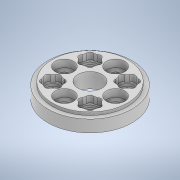
# Autodesk Inventor part: Inner_support_stand
Saved by Autodesk Inventor 2020 (Build 240168000, 168)
## iProperties
Created: 2021-09-25
Part Number: Inner_support_stand
Material: アルミニウム 2014-T4
Document SubType Name: Modeling
Designer: Masato Kubotera
Density: 2.8 g/cm^3
Appearance: 滑らか - 淡い灰色
Mass: 5.51581 g
Surface Area: 21.3058 cm^2
Volume: 1.96993 cm^3
Description: A2017 T5
Author: Masato Kubotera
Autodesk Inventor part; units mm, degrees
ref_plane "YZ Plane" through (0, 0, 0) normal (1, 0, 0) x (0, 1, 0)
ref_plane "XZ Plane" through (0, 0, 0) normal (0, 1, 0) x (-1, 0, 0)
ref_plane "XY Plane" through (0, 0, 0) normal (0, 0, 1) x (1, 0, 0)
derived "Inner_flange.ipt"
sketch "スケッチ1" plane through (0, 0, 0) normal (0, 0, 1) x (1, 0, 0)
  circle A0 centre (0, 0) radius 13.95
  line L0 (0, 13.95) -> (0, -13.95) construction
  circle A1 centre (0, 8.5) radius 1.35
  circle A2 centre (-8.5, 0) radius 1.35
  circle A3 centre (0, -8.5) radius 1.35
  circle A4 centre (8.5, 0) radius 1.35
  circle A5 centre (0, 0) radius 5 construction
  circle A6 centre (0, 0) radius 5.01
  circle A7 centre (-6.1872, 6.1872) radius 2.25
  line L1 (-9.8641, 9.8641) -> (9.8641, -9.8641) construction
  circle A8 centre (-6.1872, 6.1872) radius 1.55
  line L2 (-9.2656, 5.3623) -> (-8.9938, 6.3766) construction
  line L3 (-8.4407, 8.4407) -> (-7.4265, 8.7125) construction
  line L4 (-5.3623, 9.2656) -> (-4.6199, 8.5231) construction
  line L5 (-3.1088, 7.012) -> (-3.3806, 5.9978) construction
  line L6 (-3.9337, 3.9337) -> (-4.9479, 3.6619) construction
  line L7 (-7.012, 3.1088) -> (-7.7545, 3.8513) construction
  circle A9 centre (0, 0) radius 12.49
  arc A10 (-7.4265, 8.7125) -> (-8.7125, 7.4265) centre (-7.6983, 7.6983) ccw
  arc A11 (-8.9938, 6.3766) -> (-8.5231, 4.6199) centre (-8.2513, 5.6341) ccw
  arc A12 (-7.7545, 3.8513) -> (-5.9978, 3.3806) centre (-6.7403, 4.123) ccw
  arc A13 (-4.9479, 3.6619) -> (-3.6619, 4.9479) centre (-4.6761, 4.6761) ccw
  arc A14 (-3.3806, 5.9978) -> (-3.8513, 7.7545) centre (-4.123, 6.7403) ccw
  arc A15 (-4.6199, 8.5231) -> (-6.3766, 8.9938) centre (-5.6341, 8.2513) ccw
  line L8 (-6.3766, 8.9938) -> (-5.3623, 9.2656) construction
  line L9 (-7.4265, 8.7125) -> (-6.3766, 8.9938)
  line L10 (-4.6199, 8.5231) -> (-3.8513, 7.7545)
  line L11 (-3.8513, 7.7545) -> (-3.1088, 7.012) construction
  line L12 (-3.3806, 5.9978) -> (-3.6619, 4.9479)
  line L13 (-3.6619, 4.9479) -> (-3.9337, 3.9337) construction
  line L14 (-4.9479, 3.6619) -> (-5.9978, 3.3806)
  line L15 (-5.9978, 3.3806) -> (-7.012, 3.1088) construction
  line L16 (-7.7545, 3.8513) -> (-8.5231, 4.6199)
  line L17 (-8.5231, 4.6199) -> (-9.2656, 5.3623) construction
  line L18 (-8.9938, 6.3766) -> (-8.7125, 7.4265)
  line L19 (-8.7125, 7.4265) -> (-8.4407, 8.4407) construction
  circle A16 centre (-8.5, 0) radius 3.05
  line L20 (-8.7125, -7.4265) -> (-8.9938, -6.3766)
  circle A17 centre (-6.1872, -6.1872) radius 2.25
  circle A18 centre (-6.1872, -6.1872) radius 1.55
  circle A19 centre (0, -8.5) radius 3.05
  arc A20 (-3.8513, -7.7545) -> (-3.3806, -5.9978) centre (-4.123, -6.7403) ccw
  line L21 (-3.6619, -4.9479) -> (-3.3806, -5.9978)
  arc A21 (-3.6619, -4.9479) -> (-4.9479, -3.6619) centre (-4.6761, -4.6761) ccw
  line L22 (-5.9978, -3.3806) -> (-4.9479, -3.6619)
  arc A22 (-5.9978, -3.3806) -> (-7.7545, -3.8513) centre (-6.7403, -4.123) ccw
  line L23 (-8.5231, -4.6199) -> (-7.7545, -3.8513)
  arc A23 (-8.5231, -4.6199) -> (-8.9938, -6.3766) centre (-8.2513, -5.6341) ccw
  arc A24 (-8.7125, -7.4265) -> (-7.4265, -8.7125) centre (-7.6983, -7.6983) ccw
  line L24 (-6.3766, -8.9938) -> (-7.4265, -8.7125)
  arc A25 (-6.3766, -8.9938) -> (-4.6199, -8.5231) centre (-5.6341, -8.2513) ccw
  line L25 (-3.8513, -7.7545) -> (-4.6199, -8.5231)
  line L26 (7.4265, -8.7125) -> (6.3766, -8.9938)
  circle A26 centre (6.1872, -6.1872) radius 2.25
  circle A27 centre (6.1872, -6.1872) radius 1.55
  circle A28 centre (8.5, 0) radius 3.05
  arc A29 (7.7545, -3.8513) -> (5.9978, -3.3806) centre (6.7403, -4.123) ccw
  line L27 (4.9479, -3.6619) -> (5.9978, -3.3806)
  arc A30 (4.9479, -3.6619) -> (3.6619, -4.9479) centre (4.6761, -4.6761) ccw
  line L28 (3.3806, -5.9978) -> (3.6619, -4.9479)
  arc A31 (3.3806, -5.9978) -> (3.8513, -7.7545) centre (4.123, -6.7403) ccw
  line L29 (4.6199, -8.5231) -> (3.8513, -7.7545)
  arc A32 (4.6199, -8.5231) -> (6.3766, -8.9938) centre (5.6341, -8.2513) ccw
  arc A33 (7.4265, -8.7125) -> (8.7125, -7.4265) centre (7.6983, -7.6983) ccw
  line L30 (8.9938, -6.3766) -> (8.7125, -7.4265)
  arc A34 (8.9938, -6.3766) -> (8.5231, -4.6199) centre (8.2513, -5.6341) ccw
  line L31 (7.7545, -3.8513) -> (8.5231, -4.6199)
  line L32 (8.7125, 7.4265) -> (8.9938, 6.3766)
  circle A35 centre (6.1872, 6.1872) radius 2.25
  circle A36 centre (6.1872, 6.1872) radius 1.55
  circle A37 centre (0, 8.5) radius 3.05
  arc A38 (3.8513, 7.7545) -> (3.3806, 5.9978) centre (4.123, 6.7403) ccw
  line L33 (3.6619, 4.9479) -> (3.3806, 5.9978)
  arc A39 (3.6619, 4.9479) -> (4.9479, 3.6619) centre (4.6761, 4.6761) ccw
  line L34 (5.9978, 3.3806) -> (4.9479, 3.6619)
  arc A40 (5.9978, 3.3806) -> (7.7545, 3.8513) centre (6.7403, 4.123) ccw
  line L35 (8.5231, 4.6199) -> (7.7545, 3.8513)
  arc A41 (8.5231, 4.6199) -> (8.9938, 6.3766) centre (8.2513, 5.6341) ccw
  arc A42 (8.7125, 7.4265) -> (7.4265, 8.7125) centre (7.6983, 7.6983) ccw
  line L36 (6.3766, 8.9938) -> (7.4265, 8.7125)
  arc A43 (6.3766, 8.9938) -> (4.6199, 8.5231) centre (5.6341, 8.2513) ccw
  line L37 (3.8513, 7.7545) -> (4.6199, 8.5231)
  line L38 (-8.8318, 8.8318) -> (-3.5426, 3.5426) construction
  circle A44 centre (0, 0) radius 4
  point P0 (-7.012, 3.1088)
  point P1 (-3.9337, 3.9337)
  point P2 (-3.1088, 7.012)
  point P3 (-3.1088, -7.012)
  point P4 (-3.9337, -3.9337)
  point P5 (-7.012, -3.1088)
  point P6 (-9.2656, -5.3623)
  point P7 (-8.4407, -8.4407)
  point P8 (-5.3623, -9.2656)
  point P9 (7.012, -3.1088)
  point P10 (3.9337, -3.9337)
  point P11 (3.1088, -7.012)
  point P12 (5.3623, -9.2656)
  point P13 (8.4407, -8.4407)
  point P14 (9.2656, -5.3623)
  point P15 (3.1088, 7.012)
  point P16 (3.9337, 3.9337)
  point P17 (7.012, 3.1088)
  point P18 (9.2656, 5.3623)
  point P19 (8.4407, 8.4407)
  point P20 (5.3623, 9.2656)
  point P21 (-9.2318, 8.3532)
  point P22 (-9.2318, -8.3532)
  point P23 (-8.3532, -9.2318)
  point P24 (8.3532, -9.2318)
  point P25 (9.2318, -8.3532)
  point P26 (9.2318, 8.3532)
  point P27 (8.3532, 9.2318)
  point P28 (-8.3532, 9.2318)
  dimension "d37" = 24.98
  dimension "d3" = 4.5
  dimension "d4" = 45
  dimension "d6" = 10
  dimension "d26" = 3.1
  dimension "d38" = 1.05
  dimension "d41" = 360
  dimension "d43" = 5.52
  dimension "d44" = 6.1
  dimension "d47" = 360
  dimension "d50" = 8
  measures "d3" diameter of A7
  measures "d4" angle of L1 L0
  measures "d6" diameter of A5
  measures "d26" diameter of A8
  measures "d38" radius of A10
  measures "d43" distance between parallel lines of L12 L18
  measures "d44" diameter of A16
  measures "d50" diameter of A44
extrude "押し出し1" add sketch "スケッチ1" along normal blind 5 contours A6 | A9
extrude "押し出し2" add sketch "スケッチ1" along normal blind 4 contours A0
extrude "押し出し3" add sketch "スケッチ1" along normal blind 2.8 contours L9 A15 L10 A14 L12 A13 L14 A12 L16 A11 L18 A10 | L20 A23 L23 A22 L22 A21 L21 A20 L25 A25 L24 A24 | L26 A32 L29 A31 L28 A30 L27 A29 L31 A34 L30 A33 | L32 A41 L35 A40 L34 A39 L33 A38 L37 A43 L36 A42
extrude "押し出し4" add sketch "スケッチ1" along normal blind 2 contours A7 | A17 | A26 | A35
extrude "押し出し5" add sketch "スケッチ1" along normal blind 2.5 contours A16 | A19 | A28 | A37
